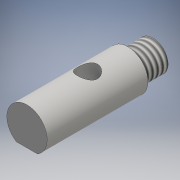
# Autodesk Inventor part: shaftcranp
Saved by Autodesk Inventor 2016 SP1 (Build 200210100, 210)
## iProperties
Created: 2017-01-23
Part Number: shaftcranp
Material: 一般
Document SubType Name: Modeling
Designer: p_admin
Density: 1 g/cm^3
Appearance: 既定
Author: p_admin
Autodesk Inventor part; units mm, degrees
ref_plane "YZ Plane" through (0, 0, 0) normal (1, 0, 0) x (0, 1, 0)
ref_plane "XZ Plane" through (0, 0, 0) normal (0, 1, 0) x (-1, 0, 0)
ref_plane "XY Plane" through (0, 0, 0) normal (0, 0, 1) x (1, 0, 0)
sketch "スケッチ1" plane through (0, 0, 0) normal (0, 1, 0) x (-1, 0, 0)
  circle A0 centre (0, 0) radius 1.5
  dimension "d0" = 3
  constraints: 1 centre point, 1 coincident
  measures "d0" diameter of A0
extrude "押し出し1" add sketch "スケッチ1" along normal blind 2.5
thread "ねじ1" size "M3x0.5" class "6g" standard "ANSI Metric M Profile" full length
sketch "スケッチ2" plane through (0, 0, 0) normal (0, -1, 0) x (1, 0, 0)
  circle A0 centre (0, 0) radius 2
  line L0 (0, -2) -> (0, -1.7)
  line L1 (0, -1.7) -> (-1.0536, -1.7)
  line L2 (0, -1.7) -> (1.0536, -1.7)
  dimension "d5" = 4
  dimension "d6" = 0.3
  constraints: 6 end point, 3 point on circle, 1 centre point, 1 coincident, 1 perpendicular, 1 point on line, 1 vertical
  measures "d5" diameter of A0
  measures "d6" distance of L0.start L0.end
extrude "押し出し2" add sketch "スケッチ2" along normal blind 10 contours A0 L2 L1
sketch "スケッチ3" plane through (1.0536, 0, -1.7) normal (0, 0, -1) x (-1, 0, 0)
  circle A0 centre (1.0536, -4) radius 1
  line L0 (2.1071, 0) -> (0, 0) projected
  point P0 (1.0536, 0)
  dimension "d9" = 2
  dimension "d10" = 4
  constraints: 1 centre point
  measures "d9" diameter of A0
  measures "d10" distance from line of L0 A0.centre
extrude "押し出し3" cut sketch "スケッチ3" against normal blind 10
